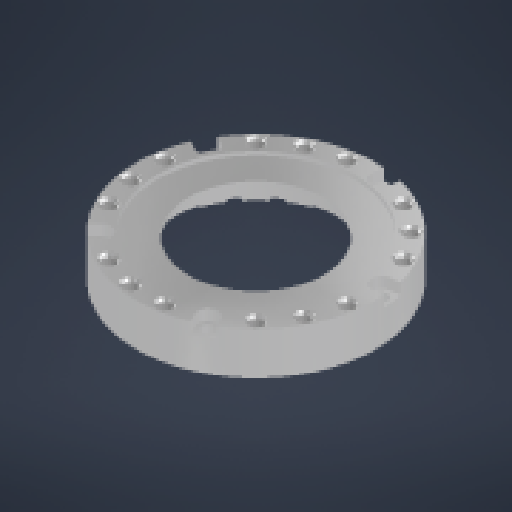
# Autodesk Inventor part: Case_GB
Saved by Autodesk Inventor 2024.2 (Build 282272000, 272)
## iProperties
Created: 2026-01-04
Part Number: Case_GB
Material: Aluminum 6061
Document SubType Name: Modeling
Designer: 4aida
Density: 2.7 g/cm^3
Appearance: Aluminum - Flat
Author: 4aida
Autodesk Inventor part; units mm, degrees
ref_plane "YZ Plane" through (0, 0, 0) normal (1, 0, 0) x (0, 1, 0)
ref_plane "XZ Plane" through (0, 0, 0) normal (0, 1, 0) x (-1, 0, 0)
ref_plane "XY Plane" through (0, 0, 0) normal (0, 0, 1) x (1, 0, 0)
sketch "Sketch1" plane through (0, 0, 0) normal (0, 0, 1) x (1, 0, 0)
  line L0 (0, 7.6) -> (0, -7.6)
  line L1 (42.5, -7.6) -> (42.5, 7.6)
  line L2 (42.5, 7.6) -> (24, 7.6)
  line L3 (24, 7.6) -> (24, 4.6)
  line L4 (24, 4.6) -> (29, 4.6)
  line L5 (29, 4.6) -> (29, -2.4)
  line L6 (29, -2.4) -> (35, -2.4)
  line L7 (35, -2.4) -> (35, -7.6)
  line L8 (35, -7.6) -> (42.5, -7.6)
  point P0 (0, 0)
  point P1 (0, 0)
  dimension "d0" = 58
  dimension "d1" = 7
  dimension "d2" = 48
  dimension "d3" = 3
  dimension "d4" = 5.2
  dimension "d5" = 70
  dimension "d6" = 85
  constraints: 18 end point, 7 perpendicular, 2 horizontal alignment, 2 vertical, 1 coincident, 1 midpoint
  measures "d0" diameter of L5 L0
  measures "d1" distance of L4.end L5.end
  measures "d2" diameter of L3 L0
  measures "d3" distance of L2.end L3.end
  measures "d4" distance between parallel lines of L8 L6
  measures "d5" diameter of L7 L0
  measures "d6" diameter of L1 L0
revolve "Revolution1" add sketch "Sketch1" angle 360 about axis through (0, 7.6, 0) along (0, -1, 0)
sketch "Sketch2" plane through (0, -7.6, 0) normal (0, -1, 0) x (1, 0, 0)
  point P0 (0, 0)
  point P1 (-35, 0)
  dimension "d8" = 35
  constraints: 1 horizontal alignment
  measures "d8" distance of point (0, 0) point (-35, 0)
hole "Hole1" at (-35, -7.6, 0) direction (0, 1, 0) diameter 4 depth 10 tip angle 118
pattern_circular "Circular Pattern1" count 20 over 360 about axis through (0, -5, 0) along (0, -1, 0) of "Hole1"
sketch "Sketch3" plane through (0, 7.6, 0) normal (0, 1, 0) x (1, 0, 0)
  arc A0 (-33.8504, -8.8966) -> (-32.6149, -12.6993) centre (-33.287, -10.8156) ccw projected
  arc A1 (-32.6149, -12.6993) -> (-29.4445, -18.9215) centre (0, 0) ccw projected
  arc A2 (-29.4445, -18.9215) -> (-27.0943, -22.1563) centre (-28.3156, -20.5725) ccw projected
  arc A3 (-27.0943, -22.1563) -> (-22.1563, -27.0943) centre (0, 0) ccw projected
  arc A4 (-22.1563, -27.0943) -> (-18.9215, -29.4445) centre (-20.5725, -28.3156) ccw projected
  arc A5 (-18.9215, -29.4445) -> (-12.6993, -32.6149) centre (0, 0) ccw projected
  arc A6 (-12.6993, -32.6149) -> (-8.8966, -33.8504) centre (-10.8156, -33.287) ccw projected
  arc A7 (-8.8966, -33.8504) -> (-1.9992, -34.9429) centre (0, 0) ccw projected
  arc A8 (-1.9992, -34.9429) -> (1.9992, -34.9429) centre (0, -35) ccw projected
  arc A9 (1.9992, -34.9429) -> (8.8966, -33.8504) centre (0, 0) ccw projected
  arc A10 (8.8966, -33.8504) -> (12.6993, -32.6149) centre (10.8156, -33.287) ccw projected
  arc A11 (12.6993, -32.6149) -> (18.9215, -29.4445) centre (0, 0) ccw projected
  arc A12 (18.9215, -29.4445) -> (22.1563, -27.0943) centre (20.5725, -28.3156) ccw projected
  arc A13 (22.1563, -27.0943) -> (27.0943, -22.1563) centre (0, 0) ccw projected
  arc A14 (27.0943, -22.1563) -> (29.4445, -18.9215) centre (28.3156, -20.5725) ccw projected
  arc A15 (29.4445, -18.9215) -> (32.6149, -12.6993) centre (0, 0) ccw projected
  arc A16 (32.6149, -12.6993) -> (33.8504, -8.8966) centre (33.287, -10.8156) ccw projected
  arc A17 (33.8504, -8.8966) -> (34.9429, -1.9992) centre (0, 0) ccw projected
  arc A18 (34.9429, -1.9992) -> (34.9429, 1.9992) centre (35, 0) ccw projected
  arc A19 (34.9429, 1.9992) -> (33.8504, 8.8966) centre (0, 0) ccw projected
  arc A20 (33.8504, 8.8966) -> (32.6149, 12.6993) centre (33.287, 10.8156) ccw projected
  arc A21 (32.6149, 12.6993) -> (29.4445, 18.9215) centre (0, 0) ccw projected
  arc A22 (29.4445, 18.9215) -> (27.0943, 22.1563) centre (28.3156, 20.5725) ccw projected
  arc A23 (27.0943, 22.1563) -> (22.1563, 27.0943) centre (0, 0) ccw projected
  arc A24 (22.1563, 27.0943) -> (18.9215, 29.4445) centre (20.5725, 28.3156) ccw projected
  arc A25 (18.9215, 29.4445) -> (12.6993, 32.6149) centre (0, 0) ccw projected
  arc A26 (12.6993, 32.6149) -> (8.8966, 33.8504) centre (10.8156, 33.287) ccw projected
  arc A27 (8.8966, 33.8504) -> (1.9992, 34.9429) centre (0, 0) ccw projected
  arc A28 (1.9992, 34.9429) -> (-1.9992, 34.9429) centre (0, 35) ccw projected
  arc A29 (-1.9992, 34.9429) -> (-8.8966, 33.8504) centre (0, 0) ccw projected
  arc A30 (-8.8966, 33.8504) -> (-12.6993, 32.6149) centre (-10.8156, 33.287) ccw projected
  arc A31 (-12.6993, 32.6149) -> (-18.9215, 29.4445) centre (0, 0) ccw projected
  arc A32 (-18.9215, 29.4445) -> (-22.1563, 27.0943) centre (-20.5725, 28.3156) ccw projected
  arc A33 (-22.1563, 27.0943) -> (-27.0943, 22.1563) centre (0, 0) ccw projected
  arc A34 (-27.0943, 22.1563) -> (-29.4445, 18.9215) centre (-28.3156, 20.5725) ccw projected
  arc A35 (-29.4445, 18.9215) -> (-32.6149, 12.6993) centre (0, 0) ccw projected
  arc A36 (-32.6149, 12.6993) -> (-33.8504, 8.8966) centre (-33.287, 10.8156) ccw projected
  arc A37 (-33.8504, 8.8966) -> (-34.9429, 1.9992) centre (0, 0) ccw projected
  arc A38 (-34.9429, 1.9992) -> (-34.9429, -1.9992) centre (-35, 0) ccw projected
  arc A39 (-34.9429, -1.9992) -> (-33.8504, -8.8966) centre (0, 0) ccw projected
  circle A40 centre (0, 0) radius 42.5 projected
  arc A41 (37.9723, 9.5579) -> (39.0674, 2.644) centre (38.5198, 6.1009) ccw
  circle A42 centre (0, 0) radius 42.5 projected
  line L0 (38.5198, 6.1009) -> (0, 0)
  line L1 (0, 0) -> (35, 0)
  line L2 (42.3817, 3.169) -> (39.0674, 2.644)
  line L3 (41.2866, 10.0828) -> (37.9723, 9.5579)
  line L4 (10.0828, 41.2866) -> (9.5579, 37.9723)
  arc A43 (2.644, 39.0674) -> (9.5579, 37.9723) centre (6.1009, 38.5198) ccw
  line L5 (3.169, 42.3817) -> (2.644, 39.0674)
  line L6 (-36.1502, 22.3476) -> (-33.1603, 20.8242)
  arc A44 (-36.3382, 14.5871) -> (-33.1603, 20.8242) centre (-34.7493, 17.7056) ccw
  line L7 (-39.3281, 16.1105) -> (-36.3382, 14.5871)
  line L8 (-32.4248, -27.4751) -> (-30.052, -25.1023)
  arc A45 (-25.1023, -30.052) -> (-30.052, -25.1023) centre (-27.5772, -27.5772) ccw
  line L9 (-27.4751, -32.4248) -> (-25.1023, -30.052)
  line L10 (16.1105, -39.3281) -> (14.5871, -36.3382)
  arc A46 (20.8242, -33.1603) -> (14.5871, -36.3382) centre (17.7056, -34.7493) ccw
  line L11 (22.3476, -36.1502) -> (20.8242, -33.1603)
  point P0 (0, 0)
  dimension "d19" = 7
  dimension "d24" = 9
  dimension "d27" = 360
  constraints: 24 end point, 10 point on circle, 5 centre point, 2 symmetric about line, 1 horizontal, 1 parallel, 1 tangent, 44 other
  measures "d19" diameter of A41
  measures "d24" angle of L1 L0
extrude "Extrusion1" cut sketch "Sketch3" against normal blind 4 contours L2 A41 L3 A40 | A40 L10 A46 L11 | L4 A43 L5 A40 | A40 L8 A45 L9 | L6 A44 L7 A40
sketch "Sketch4" plane through (0, 3.6, 0) normal (0, 1, 0) x (1, 0, 0)
  arc A0 (2.644, 39.0674) -> (9.5579, 37.9723) centre (6.1009, 38.5198) ccw projected
  point P0 (0, 0)
  constraints: 1 coincident
hole "Hole2" at (6.1009, 3.6, -38.5198) direction (0, -1, 0) diameter 4.2 end through all
pattern_circular "Circular Pattern2" count 5 over 360 about axis through (0, 6.1, 0) along (0, -1, 0) of "Hole2"
sketch "Sketch5" plane through (0, 7.6, 0) normal (0, 1, 0) x (0.9876883, 0, 0.1564345)
  circle A0 centre (22.9236, -31.5517) radius 2.1 projected
  circle A1 centre (0, 0) radius 29 projected
  point P0 (0, 0)
  point P1 (31.5517, -22.9236)
  point P2 (37.0912, -12.0517)
  point P3 (39, 0)
  point P4 (37.0912, 12.0517)
  point P5 (31.5517, 22.9236)
  point P6 (22.9236, 31.5517)
  point P7 (12.0517, 37.0912)
  point P8 (0, 39)
  point P9 (-12.0517, 37.0912)
  point P10 (-22.9236, 31.5517)
  point P11 (-31.5517, 22.9236)
  point P12 (-37.0912, 12.0517)
  point P13 (-39, 0)
  point P14 (-37.0912, -12.0517)
  point P15 (-31.5517, -22.9236)
  point P16 (-22.9236, -31.5517)
  point P17 (-12.0517, -37.0912)
  point P18 (0, -39)
  point P19 (12.0517, -37.0912)
  dimension "d43" = 360
  constraints: 1 coincident, 21 other
hole "Hole3" at (27.5772, 7.6, 27.5772) at (34.7493, 7.6, 17.7056) at (38.5198, 7.6, 6.1009) at (34.7493, 7.6, -17.7056) at (27.5772, 7.6, -27.5772) at (17.7056, 7.6, -34.7493) at (-6.1009, 7.6, -38.5198) at (-17.7056, 7.6, -34.7493) at (-27.5772, 7.6, -27.5772) at (-38.5198, 7.6, -6.1009) at (-38.5198, 7.6, 6.1009) at (-34.7493, 7.6, 17.7056) at (-17.7056, 7.6, 34.7493) at (-6.1009, 7.6, 38.5198) at (6.1009, 7.6, 38.5198) direction (0, -1, 0) diameter 4.134 depth 12 tip angle 118 countersink diameter 6 countersink angle 90 thread size "M5x0.8" class "6H" standard "ANSI Metric M Profile"
sketch "Sketch6" plane through (0, 7.6, 0) normal (0, 1, 0) x (0.9876883, 0, 0.1564345)
  circle A0 centre (0, 0) radius 25.019
  circle A1 centre (0, 0) radius 35.052
  circle A2 centre (0, 0) radius 24 projected
  dimension "d52" = 50.038
  dimension "d53" = 70.104
  constraints: 2 centre point, 2 coincident
  measures "d52" diameter of A0
  measures "d53" diameter of A1
extrude "Extrusion2" cut sketch "Sketch6" against normal blind 1.5 contours A0 | A1
body "Solid1"
